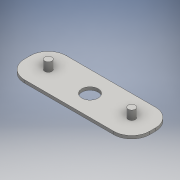
# Autodesk Inventor part: Kroller Holder2
Saved by Autodesk Inventor 2016 (Build 200138000, 138)
## iProperties
Created: 2018-03-02
Part Number: Kroller Holder2
Material: Generic
Document SubType Name: Modeling
Designer: Simon
Density: 1 g/cm^3
Appearance: Default
Author: Simon
Autodesk Inventor part; units mm, degrees
ref_plane "YZ Plane" through (0, 0, 0) normal (1, 0, 0) x (0, 1, 0)
ref_plane "XZ Plane" through (0, 0, 0) normal (0, 1, 0) x (-1, 0, 0)
ref_plane "XY Plane" through (0, 0, 0) normal (0, 0, 1) x (1, 0, 0)
sketch "Sketch1" plane through (0, 0, 0) normal (0, 0, 1) x (1, 0, 0)
  line L0 (0, 0) -> (42, 0)
  line L1 (42, 0) -> (42, 14)
  line L2 (42, 14) -> (0, 14)
  line L3 (0, 14) -> (0, 0)
  dimension "d0" = 42
  dimension "d1" = 14
  constraints: 8 end point, 2 parallel, 1 horizontal, 1 perpendicular
  measures "d0" distance of L2.end L1.end
  measures "d1" distance of L1.end L0.end
extrude "Extrusion1" add sketch "Sketch1" along normal blind 1
sketch "Sketch2" plane through (0, 0, 1) normal (0, 0, 1) x (1, 0, 0)
  line L0 (42, 14) -> (0, 14) projected
  line L1 (0, 14) -> (0, 0) projected
  circle A0 centre (7, 7) radius 1.2
  circle A1 centre (35, 7) radius 1.2
  dimension "d5" = 42
  dimension "d6" = 14
  dimension "d9" = 2.4
  dimension "d10" = 2.4
  constraints: 2 centre point
  measures "d5" distance of L0.start L0.end
  measures "d6" distance of L0.end L1.end
  measures "d9" diameter of A0
  measures "d10" diameter of A1
fillet "Fillet2" radius 6 4 edges at (42, 14, 0.5) (0, 14, 0.5) (42, 0, 0.5) (0, 0, 0.5)
extrude "Extrusion5" add sketch "Sketch2" along normal blind 3
sketch "Sketch4" plane through (0, 0, 1) normal (0, 0, 1) x (1, 0, 0)
  circle A0 centre (21, 7) radius 2.75
  line L0 (6, 0) -> (36, 0) projected
  line L1 (0, 8) -> (0, 6) projected
  circle A1 centre (7, 7) radius 1.2 projected
  point P0 (0, 0)
  dimension "d25" = 5.5
  dimension "d26" = 7
  dimension "d29" = 14
  constraints: 1 centre point
  measures "d25" diameter of A0
  measures "d26" distance from line of L0 A0.centre
  measures "d29" distance of A1.centre A0.centre
extrude "Extrusion6" cut sketch "Sketch4" against normal through all contours A0
body "Solid1"
